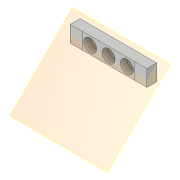
# Autodesk Inventor part: brace
Saved by Autodesk Inventor 2019 (Build 230136000, 136)
## iProperties
Created: 2016-01-06
Part Number: brace
Material: Generic
Document SubType Name: Modeling
Designer: spim
Density: 1 g/cm^3
Appearance: Default
Author: spim
Autodesk Inventor part; units mm, degrees
ref_plane "YZ Plane" through (0, 0, 0) normal (1, 0, 0) x (0, 1, 0)
ref_plane "XZ Plane" through (0, 0, 0) normal (0, 1, 0) x (-1, 0, 0)
ref_plane "XY Plane" through (0, 0, 0) normal (0, 0, 1) x (1, 0, 0)
sketch "Sketch1" plane through (0, 0, 0) normal (0, 0, 1) x (1, 0, 0)
  line L0 (-18.75, 4.0135) -> (18.75, 4.0135)
  line L1 (18.75, 4.0135) -> (18.75, -3.9865)
  line L2 (18.75, -3.9865) -> (-18.75, -3.9865)
  line L3 (-18.75, -3.9865) -> (-18.75, 4.0135)
  dimension "d0" = 8
  dimension "d1" = 37.5
  constraints: 8 end point, 2 parallel, 1 horizontal, 1 perpendicular
  measures "d0" distance of L0.end L1.end
  measures "d1" distance of L0.start L0.end
extrude "Extrusion1" add sketch "Sketch1" along normal blind 4.8
sketch "Sketch2" plane through (0, 0, 4.8) normal (0, 0, 1) x (1, 0, 0)
  line L0 (-12.7, -25.8) -> (12.7, -25.8)
  line L1 (12.7, -25.8) -> (12.7, 4.0135)
  line L2 (12.7, 4.0135) -> (-12.7, 4.0135)
  line L3 (-12.7, 4.0135) -> (-12.7, -25.8)
  line L4 (18.75, 4.0135) -> (-18.75, 4.0135) projected
  line L5 (-21.75, -25.8) -> (21.75, -25.8) projected
  point P0 (0, 0)
  point P1 (0, -25.8)
  dimension "d5" = 25.4
  constraints: 8 end point, 2 collinear, 2 parallel, 1 horizontal, 1 midpoint, 1 perpendicular, 1 vertical alignment
  measures "d5" distance of L1.end L2.end
extrude "Extrusion2" cut sketch "Sketch2" against normal blind 0.0001
ref_plane "Work Plane1" through (-18.75, 4.0135, 0) normal (0, 0.7071068, 0.7071068) x (1, 0, 0)
sketch "Sketch3" plane through (-18.75, 4.0135, 0) normal (0, 0.7071068, 0.7071068) x (1, 0, 0)
  line L0 (31.45, -3.394) -> (31.45, -9.0509) projected
  line L1 (0, 0) -> (37.5, 0) projected
  line L2 (31.45, -5.4109) -> (6.05, -5.4109)
  line L3 (6.05, -5.4109) -> (6.05, 0)
  line L4 (6.05, 0) -> (31.45, 0)
  line L5 (31.45, 0) -> (31.45, -5.4109)
  point P0 (31.45, -38.608)
  constraints: 8 end point, 2 parallel, 2 point on line, 1 horizontal, 1 perpendicular
extrude "Extrusion3" [suppressed]
sketch "Sketch6" plane through (0, 0, 4.7999) normal (0, 0, 1) x (1, 0, 0)
  line L0 (0, 0) -> (9, 0)
  line L1 (9, 0) -> (9, -18)
  line L2 (9, -18) -> (0, -18)
  line L3 (0, -18) -> (0, 0)
  line L4 (9, -18) -> (0, -18)
  line L5 (0, -18) -> (0, -9)
  line L6 (0, -9) -> (9, -9)
  line L7 (9, -9) -> (9, -18)
  line L8 (0, -18) -> (-9, -18)
  line L9 (-9, -18) -> (-9, -9)
  line L10 (-9, -9) -> (0, -9)
  line L11 (0, -9) -> (0, -18)
  line L12 (0, -9) -> (-9, -9)
  line L13 (-9, -9) -> (-9, 0)
  line L14 (-9, 0) -> (0, 0)
  line L15 (0, 0) -> (0, -9)
  line L16 (-9, 0) -> (0, 0)
  line L17 (0, 0) -> (0, 9)
  line L18 (0, 9) -> (-9, 9)
  line L19 (-9, 9) -> (-9, 0)
  line L20 (0, 9) -> (9, 9)
  line L21 (9, 9) -> (9, 0)
  line L22 (9, 0) -> (0, 0)
  line L23 (0, 0) -> (0, 9)
  line L24 (9, 9) -> (0, 9)
  line L25 (0, 9) -> (0, 18)
  line L26 (0, 18) -> (9, 18)
  line L27 (9, 18) -> (9, 9)
  line L28 (0, 18) -> (-9, 18)
  line L29 (-9, 18) -> (-9, 9)
  line L30 (-9, 9) -> (0, 9)
  line L31 (0, 9) -> (0, 18)
  point P0 (9, 0)
  dimension "d17" = 9
  dimension "d18" = 18
  dimension "d19" = 9
  dimension "d20" = 9
  dimension "d21" = 9
  dimension "d22" = 9
  dimension "d30" = 9
  constraints: 64 end point, 25 coincident, 16 parallel, 8 horizontal, 8 perpendicular, 3 point on line, 1 midpoint
  measures "d17" distance of L1.end L2.end
  measures "d18" distance of L0.end L1.end
  measures "d19" distance of L9.end L10.end
  measures "d20" distance of L17.end L16.end
  measures "d21" distance of L25.end L26.end
  measures "d22" distance of L24.end L25.end
  measures "d30" distance between parallel lines of L21 L23
hole "Hole1" at (0, 0, 4.7999) at (-9, 18, 4.7999) at (0, 18, 4.7999) at (9, 18, 4.7999) at (0, 9, 4.7999) at (-9, 9, 4.7999) at (-9, 0, 4.7999) at (9, 0, 4.7999) at (9, 9, 4.7999) at (-9, -9, 4.7999) at (0, -9, 4.7999) at (0, -18, 4.7999) at (-9, -18, 4.7999) at (9, -18, 4.7999) at (9, -9, 4.7999) direction (0, 0, -1) diameter 6.3 depth 3.1
equation "\"d18\" = 2 * d19"
equation "\"d19\" = d20"
equation "\"d20\" = d17"
equation "\"d21\" = d20"
equation "\"d22\" = d20"
equation "\"d30\" = d20"
body "Solid1"
